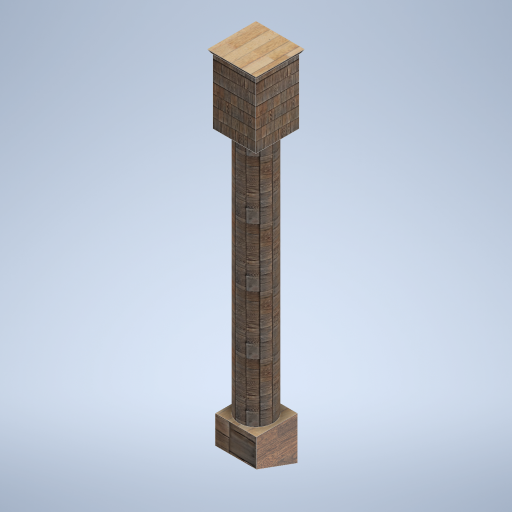
# Autodesk Inventor part: side_pillar_01
Saved by Autodesk Inventor 2024.2 (Build 282272000, 272)
## iProperties
Created: 2024-05-24
Part Number: side_pillar_01
Material: Wood (Maple)
Document SubType Name: Modeling
Designer: LOSTER_1
Density: 0.67 g/cm^3
Appearance: Natural Maple - Glossy Dark Tint
Author: LOSTER_1
Autodesk Inventor part; units mm, degrees
ref_plane "YZ Plane" through (0, 0, 0) normal (1, 0, 0) x (0, 1, 0)
ref_plane "XY Plane" through (0, 0, 0) normal (0, 0, 1) x (1, 0, 0)
sketch "Sketch1" plane through (0, 0, 0) normal (0, 1, 0) x (-1, 0, 0)
  line L0 (117.0873, -996.765) -> (117.0873, -877.765)
  line L1 (-121.9127, -877.765) -> (-121.9127, -996.765)
  line L2 (-121.9127, -1116.765) -> (-1.9127, -1116.765)
  line L3 (-2.9127, -1116.765) -> (117.0873, -1116.765)
  line L4 (117.0873, -996.765) -> (117.0873, -1116.765)
  line L5 (-121.9127, -996.765) -> (-121.9127, -1116.765)
  line L6 (117.0873, -1116.765) -> (-121.9127, -1116.765)
  line L7 (-121.9127, -1116.765) -> (-121.9127, -877.765)
  line L8 (-121.9127, -877.765) -> (117.0873, -877.765)
  line L9 (117.0873, -877.765) -> (117.0873, -1116.765)
  dimension "d0" = 239
  constraints: 20 end point, 3 perpendicular, 2 parallel, 1 horizontal
  measures "d0" distance of L1.start L2.start
ref_plane "Work Plane3" through (121.9127, 0, -1116.765) normal (-1, 0, 0) x (0, 0, 1)
ref_plane "Work Plane2" through (0, 0, 0) normal (0, 1, 0) x (-1, 0, 0)
sketch "Sketch2" plane through (121.9127, 0, -1116.765) normal (-1, 0, 0) x (0, 0, 1)
  line L0 (0, 0) -> (0, 3000)
  line L1 (239, 0) -> (239, 3000)
  line L2 (0, 0) -> (239, 86.9889)
  line L3 (0, 0) -> (254.3385, 0) construction
  line L4 (0, 0) -> (0, 250)
  line L5 (0, 250) -> (239, 250)
  line L6 (239, 250) -> (239, 86.9889)
  point P0 (1116.765, 0)
  dimension "d4" = 3000
  dimension "d5" = 3000
  dimension "d6" = 20
  dimension "d7" = 250
  constraints: 14 end point, 3 point on line, 2 perpendicular, 2 vertical, 1 equal length, 1 horizontal
  measures "d4" distance of L0.start L0.end
  measures "d5" distance of L1.start L1.end
  measures "d6" angle of L3 L2
  measures "d7" distance of L0.start L4.end
extrude "Extrusion1" add sketch "Sketch2" along normal blind 239
sketch "Sketch3" plane through (121.9127, 250, -877.765) normal (0, 1, 0) x (1, 0, 0)
  circle A0 centre (-121.9127, 119.5) radius 100
  point P0 (-121.9127, -877.765)
  dimension "d10" = 200
  constraints: 1 centre point
  measures "d10" diameter of A0
extrude "Extrusion2" add sketch "Sketch3" along normal blind 1431
sketch "Sketch4" plane through (0, 1681, -997.265) normal (0, 1, 0) x (1, 0, 0)
  line L0 (-125, -125) -> (125, -125)
  line L1 (125, -125) -> (125, 125)
  line L2 (125, 125) -> (-125, 125)
  line L3 (-125, 125) -> (-125, -125)
  line L4 (-125, -125) -> (125, 125) construction
  line L5 (125, -125) -> (-125, 125) construction
  point P0 (0, -997.265)
  point P1 (0, 0)
  point P2 (0, 0)
  point P3 (0, 0)
  dimension "d13" = 250
  dimension "d14" = 250
  constraints: 12 end point, 2 coincident, 2 midpoint, 2 parallel, 1 horizontal, 1 perpendicular
  measures "d13" distance of L2.end L1.end
  measures "d14" distance of L1.end L0.end
extrude "Extrusion3" add sketch "Sketch4" along normal blind 380
sketch "Sketch5" plane through (0, 2061, -997.265) normal (0, 1, 0) x (1, 0, 0)
  line L0 (130, -130) -> (-130, -130)
  line L1 (-130, -130) -> (-130, 130)
  line L2 (-130, 130) -> (130, 130)
  line L3 (130, 130) -> (130, -130)
  line L4 (130, -130) -> (-130, 130) construction
  line L5 (-130, -130) -> (130, 130) construction
  point P0 (0, -997.265)
  point P1 (0, 0)
  point P2 (0, 0)
  dimension "d17" = 260
  dimension "d18" = 260
  constraints: 12 end point, 2 midpoint, 2 parallel, 1 coincident, 1 horizontal, 1 perpendicular
  measures "d17" distance of L1.end L2.end
  measures "d18" distance of L0.end L1.end
extrude "Extrusion4" add sketch "Sketch5" along normal blind 20 draft 30
body "Solid1"
